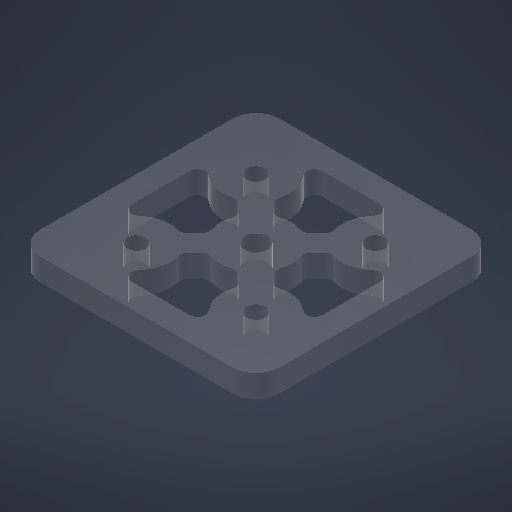
# Autodesk Inventor part: climber-axle-endcap
Saved by Autodesk Inventor 2025.1 (Build 291241020, 241B)
## iProperties
Category: _
Manager: _
Created: 2025-03-18
Part Number: climber-axle-endcap
Checked By: 00
Engr Approved By: _
User Status: Work In Process
Material: Polycarbonate, Clear
Description: SHEET METAL (mm)
Document SubType Name: Sheet Metal
Mfg Approved By: Stephen.Oerton
Designer: mathe
Manufacturer: Standard
Standards Organization: Custom
Density: 1.2 g/cm^3
Sheet Metal Rule: Default
Appearance: Polycarbonate - Clear
Mass: 10.9683 g
Surface Area: 59.6898 cm^2
Volume: 9.14021 cm^3
ILogicPurgeVersion: 2.2.20.20
OnSaveVersion: 2.2.20.20
CN_MASS: 0.0
CL_runCount: 1
CN_SERVICEABLE: _
FIRST_DESCRIPTION: _
SECOND_DESCRIPTION: _
THIRD_DESCRIPTION: _
ModelCat: Uncategorized
Subject: _
Author: mathe
Keywords: -
Revision Number: A
Autodesk Inventor part; units mm, degrees
ref_plane "YZ Plane" through (0, 0, 0) normal (1, 0, 0) x (0, 1, 0)
ref_plane "XZ Plane" through (0, 0, 0) normal (0, 1, 0) x (-1, 0, 0)
ref_plane "XY Plane" through (0, 0, 0) normal (0, 0, 1) x (1, 0, 0)
sketch "Sketch2" plane through (0, 0, 0) normal (0, 1, 0) x (-1, 0, 0)
  line L0 (45.8216, 45.8216) -> (4.9784, 45.8216)
  arc A0 (4.9784, 45.8216) -> (0, 40.8432) centre (4.9784, 40.8432) ccw
  line L1 (0, 40.8432) -> (0, 0)
  arc A1 (0, 0) -> (4.9784, -4.9784) centre (4.9784, 0) ccw
  line L2 (4.9784, -4.9784) -> (45.8216, -4.9784)
  arc A2 (45.8216, -4.9784) -> (50.8, 0) centre (45.8216, 0) ccw
  line L3 (50.8, 0) -> (50.8, 40.8432)
  arc A3 (50.8, 40.8432) -> (45.8216, 45.8216) centre (45.8216, 40.8432) ccw
  arc A4 (33.0362, 24.4657) -> (32.6118, 22.7199) centre (34.2575, 23.2444) ccw
  line L4 (33.0362, 24.4657) -> (34.4326, 25.8621)
  arc A5 (36.1326, 26.3004) -> (34.4326, 25.8621) centre (35.6539, 24.6408) ccw
  arc A6 (36.1326, 26.3004) -> (42.8397, 27.8362) centre (38.1, 33.1216) ccw
  arc A7 (45.72, 26.5503) -> (42.8397, 27.8362) centre (43.9928, 26.5503) ccw
  line L5 (45.72, 26.5503) -> (45.72, 14.2929)
  arc A8 (42.8397, 13.007) -> (45.72, 14.2929) centre (43.9928, 14.2929) ccw
  arc A9 (42.8397, 13.007) -> (36.1326, 14.5428) centre (38.1, 7.7216) ccw
  arc A10 (34.4326, 14.9811) -> (36.1326, 14.5428) centre (35.6539, 16.2024) ccw
  line L6 (34.4326, 14.9811) -> (33.0362, 16.3775)
  arc A11 (32.6118, 18.1233) -> (33.0362, 16.3775) centre (34.2575, 17.5988) ccw
  arc A12 (32.6118, 18.1233) -> (32.6118, 22.7199) centre (25.4, 20.4216) ccw
  arc A13 (17.7638, 16.3775) -> (18.1882, 18.1233) centre (16.5425, 17.5988) ccw
  line L7 (17.7638, 16.3775) -> (16.3674, 14.9811)
  arc A14 (14.6674, 14.5428) -> (16.3674, 14.9811) centre (15.1461, 16.2024) ccw
  arc A15 (14.6674, 14.5428) -> (7.9603, 13.007) centre (12.7, 7.7216) ccw
  arc A16 (5.08, 14.2929) -> (7.9603, 13.007) centre (6.8072, 14.2929) ccw
  line L8 (5.08, 14.2929) -> (5.08, 26.5503)
  arc A17 (7.9603, 27.8362) -> (5.08, 26.5503) centre (6.8072, 26.5503) ccw
  arc A18 (7.9603, 27.8362) -> (14.6674, 26.3004) centre (12.7, 33.1216) ccw
  arc A19 (16.3674, 25.8621) -> (14.6674, 26.3004) centre (15.1461, 24.6408) ccw
  line L9 (16.3674, 25.8621) -> (17.7638, 24.4657)
  arc A20 (18.1882, 22.7199) -> (17.7638, 24.4657) centre (16.5425, 23.2444) ccw
  arc A21 (18.1882, 22.7199) -> (18.1882, 18.1233) centre (25.4, 20.4216) ccw
  arc A22 (30.8405, 29.4542) -> (31.2788, 31.1542) centre (29.6192, 30.6755) ccw
  line L10 (30.8405, 29.4542) -> (29.4441, 28.0578)
  arc A23 (27.6983, 27.6334) -> (29.4441, 28.0578) centre (28.2228, 29.2791) ccw
  arc A24 (27.6983, 27.6334) -> (23.1017, 27.6334) centre (25.4, 20.4216) ccw
  arc A25 (21.3559, 28.0578) -> (23.1017, 27.6334) centre (22.5772, 29.2791) ccw
  line L11 (21.3559, 28.0578) -> (19.9595, 29.4542)
  arc A26 (19.5212, 31.1542) -> (19.9595, 29.4542) centre (21.1808, 30.6755) ccw
  arc A27 (19.5212, 31.1542) -> (17.9854, 37.8613) centre (12.7, 33.1216) ccw
  arc A28 (19.2713, 40.7416) -> (17.9854, 37.8613) centre (19.2713, 39.0144) ccw
  line L12 (19.2713, 40.7416) -> (31.5287, 40.7416)
  arc A29 (32.8146, 37.8613) -> (31.5287, 40.7416) centre (31.5287, 39.0144) ccw
  arc A30 (32.8146, 37.8613) -> (31.2788, 31.1542) centre (38.1, 33.1216) ccw
  arc A31 (19.9595, 11.389) -> (19.5212, 9.689) centre (21.1808, 10.1677) ccw
  line L13 (19.9595, 11.389) -> (21.3559, 12.7854)
  arc A32 (23.1017, 13.2098) -> (21.3559, 12.7854) centre (22.5772, 11.5641) ccw
  arc A33 (23.1017, 13.2098) -> (27.6983, 13.2098) centre (25.4, 20.4216) ccw
  arc A34 (29.4441, 12.7854) -> (27.6983, 13.2098) centre (28.2228, 11.5641) ccw
  line L14 (29.4441, 12.7854) -> (30.8405, 11.389)
  arc A35 (31.2788, 9.689) -> (30.8405, 11.389) centre (29.6192, 10.1677) ccw
  arc A36 (31.2788, 9.689) -> (32.8146, 2.9819) centre (38.1, 7.7216) ccw
  arc A37 (31.5287, 0.1016) -> (32.8146, 2.9819) centre (31.5287, 1.8288) ccw
  line L15 (31.5287, 0.1016) -> (19.2713, 0.1016)
  arc A38 (17.9854, 2.9819) -> (19.2713, 0.1016) centre (19.2713, 1.8288) ccw
  arc A39 (17.9854, 2.9819) -> (19.5212, 9.689) centre (12.7, 7.7216) ccw
  circle A40 centre (12.7, 7.7216) radius 2.0193
  circle A41 centre (12.7, 33.1216) radius 2.0193
  circle A42 centre (38.1, 33.1216) radius 2.0193
  circle A43 centre (38.1, 7.7216) radius 2.0193
  circle A44 centre (25.4, 20.4216) radius 2.4892
  point P0 (0, 40.8432)
  point P1 (4.9784, -4.9784)
  point P2 (50.8, 0)
  point P3 (23.1017, 13.2098)
  point P4 (27.6983, 13.2098)
  point P5 (29.4441, 12.7854)
  point P6 (32.8146, 2.9819)
  point P7 (31.5287, 0.1016)
  point P8 (17.9854, 2.9819)
  point P9 (19.5212, 9.689)
  point P10 (19.5212, 31.1542)
  point P11 (7.9603, 13.007)
  point P12 (5.08, 14.2929)
  point P13 (7.9603, 27.8362)
  point P14 (14.6674, 26.3004)
  point P15 (36.1326, 26.3004)
  point P16 (42.8397, 13.007)
  point P17 (36.1326, 14.5428)
  point P18 (34.4326, 14.9811)
extrude "Plate2" add sketch "Sketch2" along normal blind 4.7625
equation "\"d11\" = Thickness"
equation "\"BendRadius\" = 1.5 * Thickness"
equation "\"BendReliefWidth\" = Thickness"
equation "\"BendReliefDepth\" = 0.5 * Thickness"
equation "\"CornerReliefSize\" = 4 * Thickness"
equation "\"MinimumRemnant\" = 2 * Thickness"
equation "\"TransitionRadius\" = BendRadius"
equation "\"JacobiRadiusSize\" = BendRadius"
equation "\"GapSize\" = Thickness"
equation "\"Thickness\" = 4.7625"
body "Solid2"
